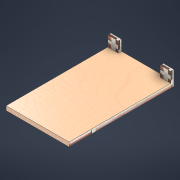
# Autodesk Inventor part: 110033226_ipt_42_城堡門口橋
Saved by Autodesk Inventor 2022 (Build 260153000, 153)
## iProperties
Created: 2022-06-26
Part Number: 110033226_ipt_42_城堡門口橋
Material: 一般
Document SubType Name: Modeling
Designer: User
Density: 1 g/cm^3
Appearance: 預設
Author: User
Autodesk Inventor part; units mm, degrees
ref_plane "YZ Plane" through (0, 0, 0) normal (1, 0, 0) x (0, 1, 0)
ref_plane "XZ Plane" through (0, 0, 0) normal (0, 1, 0) x (-1, 0, 0)
ref_plane "XY Plane" through (0, 0, 0) normal (0, 0, 1) x (1, 0, 0)
sketch "草圖1" plane through (0, 0, 0) normal (0, 0, 1) x (1, 0, 0)
  line L0 (0, 0) -> (10, 0)
  line L1 (10, 0) -> (10, 10)
  line L2 (10, 10) -> (0, 10)
  line L3 (0, 10) -> (0, 0)
  circle A0 centre (5, 5) radius 1.5
  point P0 (5, 10)
  point P1 (10, 5)
  dimension "d0" = 10
  dimension "d1" = 10
  dimension "d2" = 3
  constraints: 8 end point, 2 midpoint, 2 parallel, 1 centre point, 1 horizontal, 1 horizontal alignment, 1 perpendicular, 1 vertical alignment
  measures "d0" distance of L2.end L1.end
  measures "d1" distance of L1.end L0.end
  measures "d2" diameter of A0
extrude "擠出1" add sketch "草圖1" along normal blind 3 contours L3 L2 L1 L0 | A0
extrude "擠出2" cut sketch "草圖1" along normal blind 1.5 contours A0
sketch "草圖2" plane through (0, 0, 0) normal (0, 1, 0) x (-1, 0, 0)
  line L0 (0, 0) -> (-60, 0)
  line L1 (-60, 0) -> (-60, 100)
  line L2 (-60, 100) -> (0, 100)
  line L3 (0, 100) -> (0, 0)
  dimension "d7" = 60
  dimension "d8" = 100
  constraints: 8 end point, 2 parallel, 1 horizontal, 1 perpendicular
  measures "d7" distance of L1.end L2.end
  measures "d8" distance of L0.end L1.end
pattern_linear "矩形陣列1" count 2 spacing 50 along (1, 0, 0) of "擠出2", "擠出1"
extrude "擠出3" add sketch "草圖2" against normal blind 4
